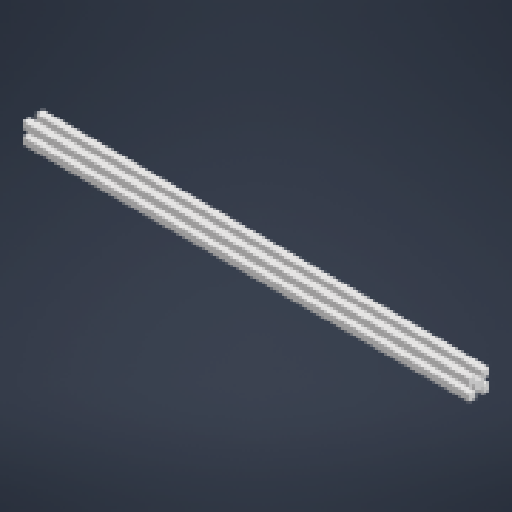
# Autodesk Inventor part: xbar
Saved by Autodesk Inventor 2025.1 (Build 291241020, 241B)
## iProperties
Created: 2024-09-23
Part Number: xbar
Material: Generic
Document SubType Name: Modeling
Designer: techn
Density: 1 g/cm^3
Appearance: Default
Author: techn
Autodesk Inventor part; units mm, degrees
ref_plane "YZ Plane" through (0, 0, 0) normal (1, 0, 0) x (0, 1, 0)
ref_plane "XZ Plane" through (0, 0, 0) normal (0, 1, 0) x (-1, 0, 0)
ref_plane "XY Plane" through (0, 0, 0) normal (0, 0, 1) x (1, 0, 0)
sketch "Sketch8" plane through (0, 0, 0) normal (0, 0, 1) x (1, 0, 0)
  line L0 (-3, 0) -> (-3, 3)
  line L1 (0, 0) -> (444, 0)
  line L2 (444, 0) -> (444, 3)
  line L3 (0, 3) -> (444, 3)
  line L4 (0, 0) -> (0, 3)
  line L5 (0, 3) -> (-3, 3)
  line L6 (0, 0) -> (-3, 0)
  line L7 (447, 3) -> (444, 3)
  line L8 (447, 0) -> (447, 3)
  line L9 (447, 0) -> (444, 0)
  line L10 (0, 4.5) -> (442, 4.5)
  line L11 (0, -1.5) -> (442, -1.5)
  line L12 (442, 4.5) -> (442, -1.5)
  line L13 (2, 4.5) -> (2, -1.5)
  line L14 (2, 4.5) -> (442, 4.5)
  line L15 (442, 4.5) -> (442, 11.5)
  line L16 (442, 11.5) -> (2, 11.5)
  line L17 (2, 11.5) -> (2, 4.5)
  line L18 (2, -1.5) -> (442, -1.5)
  line L19 (442, -1.5) -> (442, -8.5)
  line L20 (442, -8.5) -> (2, -8.5)
  line L21 (2, -8.5) -> (2, -1.5)
  point P0 (-3, 1.5)
extrude "Extrusion7" add sketch "Sketch8" along normal blind 6 contours L11 L19 L20 L21 | L17 L16 L15 L10
sketch "Sketch9" plane through (0, 0, 6) normal (0, 0, 1) x (1, 0, 0)
  line L0 (2, 11.5) -> (2, 4.5) projected
  line L1 (2, 4.5) -> (442, 4.5) projected
  line L2 (442, 4.5) -> (442, 11.5) projected
  line L3 (442, 11.5) -> (2, 11.5) projected
  line L4 (442, -8.5) -> (442, -1.5) projected
  line L5 (442, -1.5) -> (2, -1.5) projected
  line L6 (2, -1.5) -> (2, -8.5) projected
  line L7 (2, -8.5) -> (442, -8.5) projected
  line L8 (2, 4.5) -> (2, -1.5)
  line L9 (442, -1.5) -> (442, 4.5)
  point P0 (0, 0)
  constraints: 4 end point, 1 parallel, 1 vertical
extrude "Extrusion8" add sketch "Sketch9" along normal blind 1
sketch "Sketch10" plane through (0, 0, 7) normal (0, 0, 1) x (1, 0, 0)
  line L0 (2, 4.5) -> (442, 4.5) projected
  line L1 (442, -1.5) -> (2, -1.5) projected
  line L2 (442, -2.5) -> (2, -2.5)
  line L3 (2, 5.5) -> (442, 5.5)
  line L4 (2, 5.5) -> (2, -2.5)
  line L5 (2, 11.5) -> (2, -8.5) projected
  line L6 (442, 5.5) -> (442, -2.5)
  point P0 (0, 0)
  dimension "d33" = 1
  dimension "d34" = 1
  constraints: 8 end point, 3 parallel, 1 collinear
  measures "d33" distance between parallel lines of L1 L2
  measures "d34" distance between parallel lines of L0 L3
extrude "Extrusion9" add sketch "Sketch10" along normal blind 6
sketch "Sketch11" plane through (0, 0, 13) normal (0, 0, 1) x (1, 0, 0)
  line L0 (447, 0) -> (444, 0) projected
  line L1 (2, 5.5) -> (442, 5.5) projected
  line L2 (442, 5.5) -> (442, 11.5) projected
  line L3 (442, 11.5) -> (2, 11.5) projected
  line L4 (2, 11.5) -> (2, 5.5) projected
  line L5 (442, -2.5) -> (2, -2.5) projected
  line L6 (2, -2.5) -> (2, -8.5) projected
  line L7 (2, -8.5) -> (442, -8.5) projected
  line L8 (442, -8.5) -> (442, -2.5) projected
  line L9 (442, 5.5) -> (2, 5.5) projected
  line L10 (2, 5.5) -> (2, -2.5) projected
  line L11 (2, -2.5) -> (442, -2.5) projected
  line L12 (442, -2.5) -> (442, 5.5) projected
  point P0 (0, 0)
  point P1 (2, -2.5)
extrude "Extrusion10" add sketch "Sketch11" along normal blind 1
sketch "Sketch12" plane through (0, 0, 14) normal (0, 0, 1) x (1, 0, 0)
  line L0 (442, 5.5) -> (2, 5.5) projected
  line L1 (2, 11.5) -> (2, 4.5) projected
  line L2 (442, 11.5) -> (2, 11.5) projected
  line L3 (442, 4.5) -> (442, 11.5) projected
  line L4 (2, 4.5) -> (442, 4.5) projected
  line L5 (442, -8.5) -> (442, -1.5) projected
  line L6 (2, -8.5) -> (442, -8.5) projected
  line L7 (2, -1.5) -> (2, -8.5) projected
  line L8 (442, -1.5) -> (2, -1.5) projected
  point P0 (0, 0)
extrude "Extrusion11" add sketch "Sketch12" along normal blind 6
body "Solid2"
